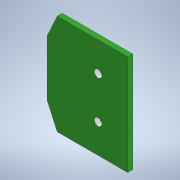
# Autodesk Inventor part: pcb
Saved by Autodesk Inventor 2022.3 (Build 263350000, 350)
## iProperties
Created: 2022-12-13
Part Number: pcb
Material: Generic
Document SubType Name: Modeling
Designer: komputer
Density: 1 g/cm^3
Appearance: Default
Author: komputer
Autodesk Inventor part; units mm, degrees
ref_plane "YZ Plane" through (0, 0, 0) normal (1, 0, 0) x (0, 1, 0)
ref_plane "XZ Plane" through (0, 0, 0) normal (0, 1, 0) x (-1, 0, 0)
ref_plane "XY Plane" through (0, 0, 0) normal (0, 0, 1) x (1, 0, 0)
sketch "Sketch1" plane through (0, 0, 0) normal (0, 0, 1) x (1, 0, 0)
  line L0 (-27.8673, 13.2738) -> (-22.4395, 22.145) projected
  line L1 (-27.3269, -6.928) -> (-27.3269, 3.472) projected
  line L2 (-20.8298, -22.6905) -> (-25.3728, -13.3353) projected
  line L3 (-7.65, -11.5) -> (7.65, -11.5) projected
  line L4 (7.65, 11.5) -> (-7.65, 11.5) projected
  arc A0 (0, 1.5) -> (0, -1.5) centre (0, 0) ccw projected
  line L5 (0, 1.5) -> (-30.65, 1.5) projected
  line L6 (-30.65, 11.5) -> (-30.65, 1.5) projected
  line L7 (-30.65, 11.5) -> (-7.65, 11.5) projected
  line L8 (-7.65, 25) -> (-7.65, 11.5) projected
  line L9 (-31.55, 25) -> (-7.65, 25) projected
  line L10 (-31.55, 25) -> (-31.55, -25) projected
  line L11 (-31.55, -25) -> (-7.65, -25) projected
  line L12 (-7.65, -11.5) -> (-7.65, -25) projected
  line L13 (-7.65, -11.5) -> (-30.65, -11.5) projected
  line L14 (-30.65, -1.5) -> (-30.65, -11.5) projected
  line L15 (-30.65, -1.5) -> (0, -1.5) projected
  line L16 (-27.3269, -1.728) -> (-27.3269, -40.6957)
  line L17 (-27.3269, -40.6957) -> (-27.3269, 31.6041)
  line L18 (-27.3269, 14.1571) -> (-22.4395, 22.145)
  line L19 (-25.3728, -13.3353) -> (-20.8298, -22.6905)
  line L20 (-25.3728, -13.3353) -> (-27.3269, -9.3114)
  line L21 (-7.65, 11.5) -> (7.65, 11.5)
  line L22 (7.65, 11.5) -> (7.65, -11.5)
  line L23 (7.65, -11.5) -> (-7.65, -11.5)
  line L24 (-7.65, -11.5) -> (-7.65, 11.5)
  line L25 (-7.65, 11.5) -> (-24.8832, 11.5)
  line L26 (-24.8832, 11.5) -> (-24.8832, -11.3233)
  line L27 (-24.8832, -11.3233) -> (-7.65, -11.3233)
  line L28 (-7.65, -11.3233) -> (-7.65, 11.5)
  line L29 (-16.2666, -11.3233) -> (-16.2666, 11.5)
  line L30 (-24.8832, -11.3233) -> (-20.8298, -20.1639)
  line L31 (-20.8298, -20.1639) -> (-9.3622, -20.1639)
  line L32 (-9.3622, -20.1639) -> (-9.3622, -11.3233)
  line L33 (-16.2666, 0.0883) -> (-13.6915, 0.0883)
  line L34 (-24.8832, 11.5) -> (-20.8298, 20.3406)
  line L35 (-20.8298, 20.3406) -> (-9.3622, 20.3406)
  line L36 (-9.3622, 20.3406) -> (-9.3622, 11.5)
  point P0 (0, 0)
  point P1 (-9.3622, -11.5)
  constraints: 42 end point, 6 point on line, 4 horizontal, 4 midpoint, 4 parallel, 3 perpendicular, 3 symmetric about line, 2 collinear, 1 vertical
extrude "Extrusion1" add sketch "Sketch1" along normal blind 2 contours L26 L5 L29 L15 | L15 L29 L27 L26 | L30 L27 L32 L13 | L13 L32 L31 L30 | L26 L7 L29 L5 | L29 L5 L24 L15 | L15 L24 L27 L29 | L32 L27 L24 L13 | L29 L7 L24 L5 | L34 L35 L36 L7 | L24 L5 A0 L15 | L15 A0 L5 L24 L4 L22 L3
sketch "Sketch2" plane through (0, 0, 2) normal (0, 0, 1) x (1, 0, 0)
  line L0 (-24.8832, -11.3233) -> (-20.8298, -20.1639) projected
  line L1 (-20.8298, -20.1639) -> (-9.3622, -20.1639) projected
  line L2 (-9.3622, -20.1639) -> (-9.3622, -11.5) projected
  line L3 (-9.3622, -11.5) -> (7.65, -11.5) projected
  line L4 (7.65, -11.5) -> (7.65, 11.5) projected
  line L5 (7.65, 11.5) -> (-9.3622, 11.5) projected
  line L6 (-9.3622, 11.5) -> (-9.3622, 20.3406) projected
  line L7 (-9.3622, 20.3406) -> (-20.8298, 20.3406) projected
  line L8 (-20.8298, 20.3406) -> (-24.8832, 11.5) projected
  line L9 (-24.8832, 11.5) -> (-24.8832, -11.3233) projected
  line L10 (-9.3622, 11.5) -> (-9.3622, 20.3406) projected
  line L11 (-9.3622, 20.3406) -> (7.65, 20.3406)
  line L12 (7.65, 20.3406) -> (7.65, -20.1639)
  line L13 (7.65, -20.1639) -> (-9.3622, -20.1639)
  line L14 (-9.3622, -20.1639) -> (-9.3622, 20.3406)
  point P0 (0, 0)
  constraints: 8 end point, 2 parallel, 1 horizontal, 1 perpendicular
extrude "Extrusion2" add sketch "Sketch2" against normal blind 2 contours L2 L3 L12 L13 | L11 L12 L5 L6
sketch "Sketch3" plane through (0, 0, 0) normal (0, 0, -1) x (-1, 0, 0)
  circle A0 centre (4.3684, -8.4591) radius 1.5 projected
  circle A1 centre (4.3684, 8.4591) radius 1.5 projected
  point P0 (0, 0)
extrude "Extrusion3" cut sketch "Sketch3" against normal blind 2
body "Solid1"
